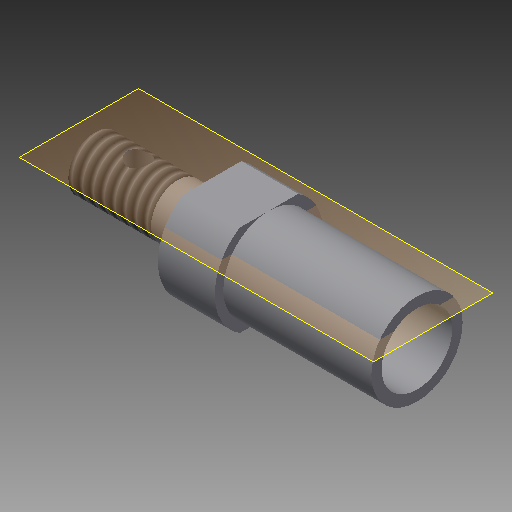
# Autodesk Inventor part: Fuel Adjuster
Saved by Autodesk Inventor 2017 (Build 210135000, 135)
## iProperties
Created: 2012-08-08
Part Number: Fuel Adjuster
Material: Generic
Document SubType Name: Modeling
Designer: John
Density: 1 g/cm^3
Appearance: Default
Author: John
Autodesk Inventor part; units mm, degrees
ref_plane "YZ Plane" through (0, 0, 0) normal (1, 0, 0) x (0, 1, 0)
ref_plane "XZ Plane" through (0, 0, 0) normal (0, 1, 0) x (-1, 0, 0)
ref_plane "XY Plane" through (0, 0, 0) normal (0, 0, 1) x (1, 0, 0)
sketch "Sketch1" plane through (0, 0, 0) normal (1, 0, 0) x (0, 1, 0)
  circle A0 centre (0, 0) radius 1.9685
  dimension "d0" = 3.937
  constraints: 1 centre point, 1 coincident
  measures "d0" diameter of A0
extrude "Extrusion1" add sketch "Sketch1" along normal blind 8.636
sketch "Sketch2" plane through (8.636, 0, 0) normal (1, 0, 0) x (0, 0, -1)
  circle A0 centre (0, 0) radius 1.9685 projected
  circle A1 centre (0, 0) radius 4.0005
  dimension "d3" = 8.001
  constraints: 1 centre point, 1 coincident
  measures "d3" diameter of A1
extrude "Extrusion2" add sketch "Sketch2" along normal blind 4.191 contours A0 | A1
sketch "Sketch3" plane through (12.827, 0, 0) normal (1, 0, 0) x (0, 0, -1)
  circle A0 centre (0, 0) radius 4.0005 projected
  circle A1 centre (0, 0) radius 3.3655
  dimension "d6" = 6.731
  constraints: 1 centre point, 1 coincident
  measures "d6" diameter of A1
extrude "Extrusion3" add sketch "Sketch3" along normal blind 10.922 contours A1
sketch "Sketch4" plane through (12.827, 0, 0) normal (1, 0, 0) x (0, 0, -1)
  circle A0 centre (0, 0) radius 3.3655 projected
  circle A1 centre (0, 0) radius 4.0005 projected
  line L0 (-3.3655, 2.1627) -> (-3.3655, -2.1627)
  line L1 (3.3655, 2.1627) -> (3.3655, -2.1627)
  constraints: 4 end point, 4 point on circle, 2 tangent, 1 parallel, 1 vertical
extrude "Extrusion4" cut sketch "Sketch4" against normal through all contours L1 A1 | L0 A1
sketch "Sketch5" plane through (23.749, 0, 0) normal (1, 0, 0) x (0, 0, -1)
  circle A0 centre (0, 0) radius 3.3655 projected
hole "Hole1" at (23.749, 0, 0) direction (-1, 0, 0) diameter 5.207 depth 5.08
sketch "Sketch6" plane through (18.669, 0, 0) normal (1, 0, 0) x (0, 0, -1)
  circle A0 centre (0, 0) radius 2.6035 projected
hole "Hole2" at (18.669, 0, 0) direction (-1, 0, 0) diameter 3.937 depth 4.953
sketch "Sketch7" plane through (13.716, 0, 0) normal (1, 0, 0) x (0, 0, -1)
  circle A0 centre (0, 0) radius 1.9685 projected
hole "Hole3" at (13.716, 0, 0) direction (-1, 0, 0) diameter 1.5748 end through all
ref_plane "Work Plane1" through (0, 0, 1.9685) normal (0, 0, 1) x (1, 0, 0)
sketch "Sketch8" plane through (0, 0, 1.9685) normal (0, 0, 1) x (1, 0, 0)
  line L0 (0, 0) -> (3.212, 0)
  constraints: 2 end point, 1 horizontal
hole "Hole4" at (3.212, 0, 1.9685) direction (0, 0, -1) diameter 1.651 depth 1.9685
thread "Thread1" size "8-32 UNC" class "2B" standard "ANSI Unified Screw Threads" full length
thread "Thread2" size "8-32 UNC" class "2A" standard "ANSI Unified Screw Threads" length 7.62 offset 2.54
body "Solid1"
